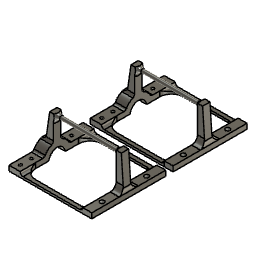
Amemometer_case v5 (Autodesk Fusion 360 design; units mm, degrees)
Autodesk Fusion 360 part; units mm, degrees
sketch "Sketch1" plane through (0, 0, 0) normal (0, 0, 1) x (1, 0, 0)
  line L0 (0.0819, -11.2497) -> (0.0819, -49.9997)
  line L1 (0.0819, -49.9997) -> (-6.9181, -49.9997)
  line L2 (-6.9181, -49.9997) -> (-6.9181, -16.9997)
  line L3 (0.0819, 11.25) -> (0.0819, 50)
  line L4 (0.0819, 50) -> (-6.9181, 50)
  line L5 (-6.9181, 50) -> (-6.9181, 17)
  line L6 (-52, -5) -> (-17.6593, -5)
  line L7 (-52, -5) -> (-52, 5)
  line L8 (-52, 5) -> (-17.6099, 5)
  arc A0 (-17.6593, -5) -> (-6.9181, -16.9997) centre (0, 0) ccw
  arc A1 (-6.9181, 17) -> (-17.6099, 5) centre (0.0819, 0) ccw
  spline S0 degree 2 poles (0.0819, -11.2497) (-52, 0) (0.0819, 11.25) knots 0 0 0 3.066333 3.066333 3.066333 weights 1 0.25 1
  dimension "d2" = 38.75
  dimension "d3" = 38.75
  dimension "d5" = 7
  dimension "d8" = 7
  dimension "d13" = 33
  dimension "d14" = 33
  dimension "d41" = 10
  dimension "d43" = 7
  dimension "d44" = 7
  dimension "d45" = 52
  dimension "d47" = 5
  dimension "d113" = 11.25
  dimension "d115" = 11.25
  constraint vertical L0
  constraint perpendicular L0 L1
  constraint perpendicular L1 L2
  constraint vertical L3
  constraint perpendicular L3 L4
  constraint perpendicular L4 L5
  constraint perpendicular L6 L7
  constraint perpendicular L2 L8
  constraint coincident A0.centre origin
  measures "d2" distance of L3.start L3.end
  measures "d3" distance of L0.start L0.end
  measures "d5" distance of L3.end L4.end
  measures "d8" distance of L0.end L1.end
  measures "d13" distance of L4.end L5.end
  measures "d14" distance of L1.end L2.end
  measures "d41" distance of L6.start L7.end
  measures "d43" horizontal distance of L2.end A1.centre
  measures "d44" horizontal distance of L5.end A1.centre
  measures "d45" distance of A0.centre L7
  measures "d47" vertical distance of A0.centre L6.start
  measures "d113" distance of A0.centre L0.start
  measures "d115" vertical distance of A0.centre L3.start
extrude "Extrude1" add sketch "Sketch1" along normal blind 15 makes body 1
sketch "Sketch2" plane through (0, -5, 0) normal (0, -1, 0) x (1, 0, 0)
  line L0 (-18.9934, 15) -> (-46, 15)
  line L1 (-52, 0) -> (-17.6593, 0)
  line L2 (-17.6593, 0) -> (-17.6593, 15)
  line L3 (-17.6593, 15) -> (-52, 15)
  line L4 (-52, 15) -> (-52, 0)
  line L5 (-17.6593, 0) -> (-52, 0)
  line L6 (-52, 10) -> (-17.6593, 5)
  dimension "d52" = 10
  dimension "d53" = 5
  constraint coincident L1.end L2.start
  constraint coincident L1.start L4.end
  constraint coincident L4 L6.start
  constraint coincident L2 L6.end
  measures "d52" distance of L1.start L6.start
  measures "d53" distance of L1.end L6.end
extrude "Extrude2" cut sketch "Sketch2" against normal blind 10 contours L1 L2 L4 L5 L6 bodies 1
fillet "Fillet1" radius 4 4 edges at (-17.6593, -5, 10) (-6.9181, -16.9997, 7.5) (-17.6099, 5, 7.5) (-6.9181, 17, 7.5) on bodies 1
fillet "Fillet2" radius 6 1 edges at (-17.6593, -0.023, 5) on bodies 1
sketch "Sketch3" plane through (0, 0, 15) normal (0, 0, 1) x (-1, 0, 0)
  line L0 (-0.0819, -11.25) -> (-0.0819, -50)
  line L1 (-0.0819, -50) -> (6.9181, -50)
  line L2 (6.9181, -50) -> (6.9181, -19.4956)
  line L3 (6.9181, 19.5057) -> (6.9181, 49.9997)
  line L4 (6.9181, 49.9997) -> (-0.0819, 49.9997)
  line L5 (-0.0819, 49.9997) -> (-0.0819, 11.2497)
  circle A0 centre (48, 0) radius 2.5
  line L6 (-0.0819, 49.9997) -> (2.9181, 49.9997)
  line L7 (2.9181, 49.9997) -> (2.9181, 44.9997)
  line L8 (2.9181, 44.9997) -> (-0.0819, 44.9997)
  line L9 (-0.0819, 44.9997) -> (-0.0819, 49.9997)
  line L10 (-0.0819, -50) -> (2.9181, -50)
  line L11 (2.9181, -50) -> (2.9181, -45)
  line L12 (2.9181, -45) -> (-0.0819, -45)
  line L13 (-0.0819, -45) -> (-0.0819, -50)
  arc A1 (8.9525, -16.0119) -> (16.7515, -7.3918) centre (-0.0819, 0) ccw
  line L14 (20.4139, -5) -> (52, -5)
  line L15 (52, -5) -> (52, 5)
  line L16 (52, 5) -> (20.4616, 5)
  arc A2 (16.8002, 7.3895) -> (8.9815, 16.0456) centre (-0.0819, 0) ccw
  arc A3 (8.9525, -16.0119) -> (6.9181, -19.4956) centre (10.9181, -19.4956) ccw
  arc A4 (20.4139, -5) -> (16.7515, -7.3918) centre (20.4139, -9) ccw
  arc A5 (16.8002, 7.3895) -> (20.4616, 5) centre (20.4616, 9) ccw
  arc A6 (6.9181, 19.5057) -> (8.9644, 16.0153) centre (10.9181, 19.5057) ccw
  spline S0 degree 2 poles (-0.0819, 11.2497) (52, 0) (-0.0819, -11.25) knots 0 0 0 3.066333 3.066333 3.066333 weights 1 0.25 1
  dimension "d35" = 5
  dimension "d36" = 3
  dimension "d37" = 5
  dimension "d38" = 5
  dimension "d39" = 3
  dimension "d50" = 4
  dimension "d51" = 5
  constraint horizontal L6
  constraint vertical L7
  constraint horizontal L8
  constraint vertical L9
  constraint coincident L4.end L5.start
  constraint horizontal L10
  constraint vertical L11
  constraint horizontal L12
  constraint vertical L13
  constraint coincident L0.end L1.start
  measures "d35" distance of L6.end L7.end
  measures "d36" distance of L7.end L8.end
  measures "d37" diameter of A0
  measures "d38" distance of L10.end L11.end
  measures "d39" distance of L11.end L12.end
  measures "d50" distance of A0.centre L15
  measures "d51" vertical distance of A0.centre L14.end
extrude "Extrude3" add sketch "Sketch3" along normal blind 85 bodies 1
sketch "Sketch4" plane through (0, 0, 100) normal (0, 0, 1) x (-1, 0, 0)
  circle A0 centre (48, 0) radius 2.5
  line L0 (0, 50) -> (0, -50)
  line L1 (0, -50) -> (7, -50)
  line L2 (7, -50) -> (7, -5)
  line L3 (7, -5) -> (52, -5)
  line L4 (52, -5) -> (52, 5)
  line L5 (52, 5) -> (7, 5)
  line L6 (7, 5) -> (7, 50)
  line L7 (7, 50) -> (0, 50)
  dimension "d103" = 10
  dimension "d104" = 45
  dimension "d105" = 45
  dimension "d106" = 100
  dimension "d107" = 7
  dimension "d108" = 7
  dimension "d109" = 50
  dimension "d110" = 7
  constraint vertical L0
  constraint perpendicular L0 L1
  constraint perpendicular L1 L2
  constraint perpendicular L0 L3
  constraint perpendicular L3 L4
  constraint perpendicular L4 L5
  constraint perpendicular L5 L6
  constraint perpendicular L6 L7
  measures "d103" distance of L3.end L4.end
  measures "d104" distance of L4.end L5.end
  measures "d105" distance of L5.end L6.end
  measures "d106" distance of L0.start L0.end
  measures "d107" distance of L0.start L6.end
  measures "d108" distance of L0.end L1.end
  measures "d109" distance of origin L0.end
  measures "d110" horizontal distance of origin L2.end
extrude "Extrude4" add sketch "Sketch4" along normal blind 12 contours A0 | L0 L1 L2 L3 L4 L5 L6 L7 bodies 1
sketch "Sketch5" plane through (0, 5, 0) normal (0, 1, 0) x (-1, 0, 0)
  line L0 (7, 100) -> (52, 100)
  line L1 (52, 100) -> (52, 112)
  line L2 (52, 112) -> (7, 112)
  line L3 (7, 112) -> (7, 100)
  line L4 (7, 112) -> (52, 112)
  line L5 (52, 107) -> (7, 110)
  dimension "d62" = 5
  dimension "d63" = 2
  constraint coincident L2.end L3.start
  constraint coincident L1.end L2.start
  constraint coincident L1 L5.start
  constraint coincident L3 L5.end
  measures "d62" distance of L1.end L5.start
  measures "d63" distance of L2.end L5.end
extrude "Extrude5" cut sketch "Sketch5" against normal blind 10 contours L1 L2 L3 L4 L5 bodies 1
fillet "Fillet3" radius 8 2 edges at (-7, 5, 105) (-7, -5, 105) on bodies 1
fillet "Fillet4" radius 8 2 edges at (-7, -4, 110) (-7, 9, 110) on bodies 1
fillet "Fillet5" radius 4 4 edges at (-2.9181, 47.5, 15) (-2.9181, -47.4997, 15) (-2.9181, 47.5, 100) (-2.9181, -47.4997, 100) on bodies 1
fillet "Fillet6" radius 16 2 edges at (-3.4181, -44.9997, 15) (-3.4181, 45, 15) on bodies 1
fillet "Fillet7" radius 8 2 edges at (-3.4591, 45, 100) (-3.4591, -44.9997, 100) on bodies 1
fillet "Fillet8" radius 6 1 edges at (-45.6692, -0.904, 15) on bodies 1
fillet "Fillet9" radius 3 1 edges at (-45.6692, 0.904, 100) on bodies 1
sketch "Sketch6" plane through (0, 0, 0) normal (1, 0, 0) x (0, 1, 0)
  circle A0 centre (42, 7.5) radius 2
  circle A1 centre (-26.9997, 7.5) radius 2
  circle A2 centre (30, 106) radius 3
  circle A3 centre (-30, 106) radius 3
  circle A4 centre (27, 7.5) radius 2
  circle A5 centre (-41.9997, 7.5) radius 2
  point P0 (50, 0)
  point P1 (-49.9997, 0)
  point P2 (50, 112)
  point P3 (-50, 112)
  dimension "d78" = 4
  dimension "d79" = 4
  dimension "d80" = 6
  dimension "d81" = 6
  dimension "d82" = 4
  dimension "d83" = 4
  dimension "d88" = 7.5
  dimension "d89" = 23
  dimension "d90" = 7.5
  dimension "d91" = 8
  dimension "d92" = 7.5
  dimension "d93" = 7.5
  dimension "d94" = 23
  dimension "d95" = 8
  measures "d78" diameter of A0
  measures "d79" diameter of A1
  measures "d80" diameter of A2
  measures "d81" diameter of A3
  measures "d82" diameter of A4
  measures "d83" diameter of A5
  measures "d88" vertical distance of A0.centre P0
  measures "d89" horizontal distance of A4.centre P0
  measures "d90" vertical distance of A4.centre P0
  measures "d91" horizontal distance of A0.centre P0
  measures "d92" vertical distance of A5.centre P1
  measures "d93" vertical distance of A1.centre P1
  measures "d94" horizontal distance of A1.centre P1
  measures "d95" horizontal distance of A5.centre P1
extrude "Extrude6" cut sketch "Sketch6" against normal blind 10 bodies 1
move_body "Move1" bodies 1 to x (1, 0, 0) y (0, 1, 0) z (0, 0, 1) at (-5, 0, 0)
move_body "Move2" bodies 1 to x (0, 0, -1) y (0, 1, 0) z (1, 0, 0) at (-4.9181, 0, -4.9181)
move_body "Move3" bodies 1 to x (1, 0, 0) y (0, 1, 0) z (0, 0, 1) at (10, 55, 0)
mirror "Mirror2" about plane through (0, 0, 0) normal (0, 1, 0) of bodies 1 makes body 2
